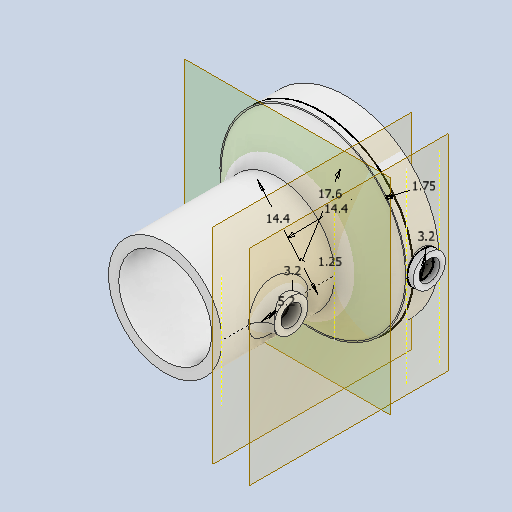
# Autodesk Inventor part: SpectroLensAdapter
Saved by Autodesk Inventor 2023 (Build 270158000, 158)
## iProperties
Created: 2022-08-19
Part Number: SpectroLensAdapter
Material: ABS Plastic
Document SubType Name: Modeling
Designer: Miner
Density: 1.06 g/cm^3
Appearance: Smooth - White
Author: Miner
Autodesk Inventor part; units mm, degrees
ref_plane "XZ Plane" through (0, 0, 0) normal (0, 1, 0) x (-1, 0, 0)
ref_plane "XY Plane" through (0, 0, 0) normal (0, 0, 1) x (1, 0, 0)
sketch "Sketch1" plane through (0, 0, 0) normal (0, 0, 1) x (1, 0, 0)
  circle A0 centre (0, 0) radius 12.75
  circle A1 centre (0, 0) radius 14.5
  dimension "d0" = 25.5
  dimension "d1" = 29
  constraints: 2 centre point, 2 coincident
  measures "d0" diameter of A0
  measures "d1" diameter of A1
extrude "Extrusion1" add sketch "Sketch1" against normal blind 4
sketch "Sketch2" plane through (0, 0, 0) normal (0, 0, 1) x (1, 0, 0)
  circle A0 centre (0, 0) radius 7.2
  circle A1 centre (0, 0) radius 8.8
  circle A2 centre (0, 0) radius 14.5
  circle A3 centre (0, 0) radius 12.75 projected
  dimension "d4" = 14.4
  dimension "d5" = 17.6
  dimension "d29" = 1.75
  constraints: 3 centre point, 3 coincident
  measures "d4" diameter of A0
  measures "d5" diameter of A1
  measures "d29" radial gap between concentric circles of A3 A2
extrude "Extrusion2" add sketch "Sketch2" along normal blind 24 contours A1
extrude "Extrusion3" add sketch "Sketch2" along normal blind 1 contours A2 | A3
chamfer "Chamfer2" distance 5.5 angle 45 1 edges at (-8.8, 0, 1)
ref_plane "Work Plane1" through (0, 0, 5) normal (0, 0, -1) x (-1, 0, 0)
sketch "Sketch3" plane through (0, 0, 5) normal (0, 0, -1) x (-1, 0, 0)
  circle A0 centre (0, 0) radius 7.2
  circle A1 centre (0, 0) radius 5.95
  dimension "d17" = 1.25
  dimension "d25" = 14.4
  constraints: 2 centre point, 1 coincident
  measures "d17" radial gap between concentric circles of A0 A1
  measures "d25" diameter of A0
extrude "Extrusion4" add sketch "Sketch3" along normal blind 1 contours A0 | A1
extrude "Extrusion5" cut sketch "Sketch3" along normal blind 1 contours A1
chamfer "Chamfer3" distance 1.25 angle 45 1 edges at (-7.2, 0, 5)
ref_plane "Work Plane2" through (14.5, 0, 0) normal (1, 0, 0) x (0, 1, 0)
sketch "Sketch4" plane through (14.5, 0, 0) normal (1, 0, 0) x (0, 1, 0)
  line L0 (-14.5, -4) -> (14.5, -4) construction
  line L1 (0, -4) -> (0, 1) construction
  line L2 (14.5, 1) -> (-14.5, 1) construction
  circle A0 centre (0, -1.5) radius 1.6
  circle A1 centre (0, -1.5) radius 2.5
  point P0 (0, 0)
  dimension "d26" = 3.2
  constraints: 3 midpoint, 2 centre point, 2 end point, 1 coincident, 1 tangent
  measures "d26" diameter of A0
extrude "Extrusion6" add sketch "Sketch4" along normal blind 1
extrude "Extrusion7" cut sketch "Sketch4" against normal blind 2 contours A0
ref_plane "Work Plane3" through (8.8, 0, 0) normal (1, 0, 0) x (0, 1, 0)
extrude "Extrusion8" add sketch "Sketch4" against normal blind 0.5
sketch "Sketch5" plane through (8.8, 0, 0) normal (1, 0, 0) x (0, 1, 0)
  line L0 (-8.8, 6.5) -> (8.8, 6.5) construction
  line L1 (0, 6.5) -> (0, 24) construction
  line L2 (8.8, 24) -> (-8.8, 24) construction
  circle A0 centre (0, 15.25) radius 1.6
  circle A1 centre (0, 15.25) radius 2.6
  point P0 (0, 0)
  dimension "d34" = 3.2
  dimension "d35" = 5.2
  constraints: 3 midpoint, 2 centre point, 2 end point, 1 coincident
  measures "d34" diameter of A0
  measures "d35" diameter of A1
extrude "Extrusion9" add sketch "Sketch5" along normal blind 2
extrude "Extrusion10" cut sketch "Sketch5" against normal blind 2 contours A0
extrude "Extrusion11" add sketch "Sketch5" against normal blind 0.5
fillet "Fillet1" radius 2 3 edges at (8.5756, 1.9745, 16.9416) (8.4071, -2.6, 15.25) (8.5756, 1.9745, 13.5584)
body "Solid1"
